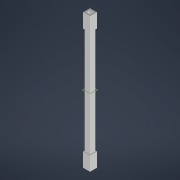
# Autodesk Inventor part: clamshell cross link
Saved by Autodesk Inventor 2021 (Build 250183000, 183)
## iProperties
Created: 2021-02-13
Part Number: clamshell cross link
Material: ABS Plastic
Document SubType Name: Modeling
Designer: vikki
Mass: 0.803536 g
Surface Area: 10.9906 cm^2
Volume: 0.758052 cm^3
Density: 1.06 g/cm^3
Appearance: Smooth - White
Author: vikki
Autodesk Inventor part; units mm, degrees
ref_plane "YZ Plane" through (0, 0, 0) normal (1, 0, 0) x (0, 1, 0)
ref_plane "XZ Plane" through (0, 0, 0) normal (0, 1, 0) x (-1, 0, 0)
ref_plane "XY Plane" through (0, 0, 0) normal (0, 0, 1) x (1, 0, 0)
sketch "Sketch1" plane through (0, 0, 0) normal (0, 1, 0) x (-1, 0, 0)
  circle A0 centre (0, 0) radius 1.15
  circle A1 centre (0, 0) radius 2
  line L0 (-2, 2) -> (2, 2)
  line L1 (2, 2) -> (2, -2)
  line L2 (2, -2) -> (-2, -2)
  line L3 (-2, -2) -> (-2, 2)
  line L4 (-2, 2) -> (2, -2) construction
  line L5 (2, 2) -> (-2, -2) construction
  dimension "d0" = 2.3
  dimension "d1" = 4
  constraints: 12 end point, 2 centre point, 2 coincident, 2 midpoint, 2 parallel, 2 tangent, 1 horizontal, 1 perpendicular
  measures "d0" diameter of A0
  measures "d1" diameter of A1
extrude "Extrusion1" add sketch "Sketch1" along normal blind 5
sketch "Sketch2" plane through (0, 5, 0) normal (0, 1, 0) x (1, 0, 0)
  line L0 (2, 2) -> (-2, 2) projected
  line L1 (-2, 2) -> (-2, -2) projected
  line L2 (-2, -2) -> (2, -2) projected
  line L3 (2, -2) -> (2, 2) projected
  circle A0 centre (0, 0) radius 1.15 projected
extrude "Extrusion2" add sketch "Sketch2" along normal blind 3 contours L3 L2 L1 L0 | A0
sketch "Sketch3" plane through (0, 8, 0) normal (0, 1, 0) x (1, 0, 0)
  line L0 (1.5, -1.5) -> (-1.5, -1.5)
  line L1 (-1.5, -1.5) -> (-1.5, 1.5)
  line L2 (-1.5, 1.5) -> (1.5, 1.5)
  line L3 (1.5, 1.5) -> (1.5, -1.5)
  line L4 (1.5, -1.5) -> (-1.5, 1.5) construction
  line L5 (-1.5, -1.5) -> (1.5, 1.5) construction
  point P0 (0, 0)
  dimension "d6" = 3
  constraints: 12 end point, 2 midpoint, 2 parallel, 2 perpendicular, 1 horizontal
  measures "d6" distance of L1.end L2.end
extrude "Extrusion3" add sketch "Sketch3" along normal blind 44.25
ref_plane "Work Plane1" through (0, 38.2, 0) normal (0, -1, 0) x (1, 0, 0)
mirror "Mirror1" about plane through (0, 38.2, 0) normal (0, -1, 0) of "Extrusion3", "Extrusion1", "Extrusion2"
body "Solid1"
